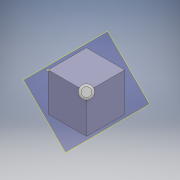
# Autodesk Inventor part: Corners
Saved by Autodesk Inventor 2018 (Build 220112000, 112)
## iProperties
Created: 2018-03-06
Part Number: Corners
Material: Generic
Document SubType Name: Modeling
Designer: sterl
Density: 1 g/cm^3
Appearance: Default
Author: sterl
Autodesk Inventor part; units mm, degrees
ref_plane "YZ Plane" through (0, 0, 0) normal (1, 0, 0) x (0, 1, 0)
ref_plane "XZ Plane" through (0, 0, 0) normal (0, 1, 0) x (-1, 0, 0)
ref_plane "XY Plane" through (0, 0, 0) normal (0, 0, 1) x (1, 0, 0)
sketch "Sketch1" plane through (0, 0, 0) normal (1, 0, 0) x (0, 1, 0)
  line L0 (0, 0) -> (10, 0)
  line L1 (0, 0) -> (0, -10)
  line L2 (10, 0) -> (10, -10)
  line L3 (10, -10) -> (0, -10)
  dimension "d0" = 10
  dimension "d1" = 10
  constraints: 8 end point, 2 vertical, 1 horizontal, 1 perpendicular
  measures "d0" distance of L0.start L0.end
  measures "d1" distance of L0.start L1.end
extrude "Extrusion1" add sketch "Sketch1" along normal blind 10
shell "Shell1" thickness 2 removed faces 3 at (3.3333, 10, -3.3333) at (3.3333, 6.6667, -10) at (0, 3.3333, -3.3333)
ref_plane "Work Plane2" through (10, 0, 0) normal (-0.5773503, 0.5773503, -0.5773503) x (0.7071068, 0, -0.7071068)
ref_plane "Work Plane1" through (0, 10, -2) normal (-0.5773503, 0.5773503, -0.5773503) x (0.7071068, 0, -0.7071068)
sketch "Sketch2" plane through (10, 0, 0) normal (-0.5773503, 0.5773503, -0.5773503) x (0.7071068, 0, -0.7071068)
  line L0 (0, -8.165) -> (0, 0) projected
  line L1 (-7.0711, 4.0825) -> (0, 0) projected
  line L2 (0, 0) -> (7.0711, 4.0825) projected
  line L3 (0, -6.532) -> (0, 0) projected
  circle A0 centre (0, 0) radius 1.5
  dimension "d5" = 3
  constraints: 1 centre point, 1 coincident
  measures "d5" diameter of A0
extrude "Extrusion2" add sketch "Sketch2" along normal up to next
sketch "Sketch3" plane through (10, 0, 0) normal (0.5773503, -0.5773503, 0.5773503) x (0.7071068, 0, -0.7071068)
  point P0 (-7.0711, -4.0825)
sketch "Sketch4" plane through (10, 0, 0) normal (0.5773503, -0.5773503, 0.5773503) x (0.7071068, 0, -0.7071068)
  circle A0 centre (0, 0) radius 1.5 projected
  point P0 (-7.0711, -4.0825)
extrude "Extrusion3" add sketch "Sketch4" along normal blind 4
fillet "Fillet1" radius 0.5 1 edges at (11.2487, -2.3094, 3.3701)
body "Solid1"
